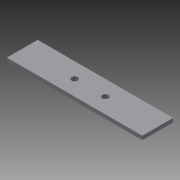
# Autodesk Inventor part: Cylinder Mount
Saved by Autodesk Inventor 2013 (Build 170138000, 138)
## iProperties
Created: 2013-01-26
Part Number: Cylinder Mount
Material: Generic
Document SubType Name: Sheet Metal
Designer: actoennies
Density: 1 g/cm^3
Sheet Metal Rule: Default
Mass: 23.7689 g
Surface Area: 175.75 cm^2
Volume: 23.7689 cm^3
Author: actoennies
Autodesk Inventor part; units mm, degrees
ref_plane "YZ Plane" through (0, 0, 0) normal (1, 0, 0) x (0, 1, 0)
ref_plane "XZ Plane" through (0, 0, 0) normal (0, 1, 0) x (-1, 0, 0)
ref_plane "XY Plane" through (0, 0, 0) normal (0, 0, 1) x (1, 0, 0)
sketch "Sketch13" plane through (0, 0, 0) normal (0, -1, 0) x (1, 0, 0)
  line L0 (0, 25.4) -> (-152.4, 25.4)
  line L1 (-152.4, 0) -> (-25.4, 0)
  line L2 (-25.4, -38.1) -> (0, -38.1)
  line L3 (-152.4, 0) -> (-152.4, -38.1)
  line L4 (-152.4, -38.1) -> (-127, -38.1)
  line L5 (-127, -38.1) -> (-127, 0)
  line L6 (-152.4, 25.4) -> (-152.4, 63.5)
  line L7 (-152.4, 63.5) -> (-127, 63.5)
  line L8 (-127, 63.5) -> (-127, 25.4)
  line L9 (0, 25.4) -> (0, 63.5)
  line L10 (0, 63.5) -> (-25.4, 63.5)
  line L11 (-25.4, 63.5) -> (-25.4, 25.4)
  circle A0 centre (-139.7, 50.8) radius 3.3782
  circle A1 centre (-139.7, -25.4) radius 3.3782
  circle A2 centre (-12.7, 50.8) radius 3.3782
  point P0 (0, 0)
  dimension "d73" = 25.4
  dimension "d74" = 38.1
  dimension "d75" = 25.4
  dimension "d76" = 38.1
  dimension "d77" = 25.4
  dimension "d78" = 6.7564
  dimension "d79" = 6.7564
  dimension "d80" = 6.7564
  dimension "d81" = 12.7
  dimension "d82" = 12.7
  dimension "d83" = 12.7
  dimension "d84" = 12.7
  dimension "d85" = 12.7
  dimension "d86" = 12.7
  dimension "d87" = 38.1
  measures "d73" distance of L3.end L4.end
  measures "d74" distance of L0.end L6.end
  measures "d75" distance of L6.end L7.end
  measures "d76" distance of L0.start L9.end
  measures "d77" distance of L9.end L10.end
  measures "d78" diameter of A0
  measures "d79" diameter of A1
  measures "d80" diameter of A2
  measures "d81" distance from line of L10 A2.centre
  measures "d82" distance from line of L9 A2.centre
  measures "d83" distance from line of L7 A0.centre
  measures "d84" distance from line of L8 A0.centre
  measures "d85" distance from line of L5 A1.centre
  measures "d86" distance from line of L4 A1.centre
  measures "d87" distance of L4.end L5.end
sketch "Sketch1" plane through (0, 0, 0) normal (0, 1, 0) x (-1, 0, 0)
  line L0 (0, 0) -> (0, 25.4)
  line L1 (0, 25.4) -> (152.4, 25.4)
  line L2 (152.4, 25.4) -> (152.4, 0)
  line L3 (152.4, 0) -> (25.4, 0)
  line L4 (0, 0) -> (0, -38.1)
  line L5 (0, -38.1) -> (25.4, -38.1)
  line L6 (25.4, -38.1) -> (25.4, 0)
  dimension "d0" = 25.4
  dimension "d1" = 152.4
  dimension "d58" = 38.1
  dimension "d59" = 25.4
  constraints: 14 end point, 4 perpendicular, 2 parallel, 1 vertical
  measures "d0" distance of L0.start L0.end
  measures "d1" distance of L0.end L1.end
  measures "d58" distance of L0.start L4.end
  measures "d59" distance of L4.end L5.end
extrude "Plate1" add sketch "Sketch1" along normal blind 3.175
sketch "Sketch5" plane through (0, 0, 0) normal (0, -1, 0) x (1, 0, 0)
  line L0 (0, 25.4) -> (-152.4, 25.4) projected
  line L1 (-152.4, 0) -> (-25.4, 0) projected
  circle A0 centre (-68.58, 12.7) radius 2.54
  circle A1 centre (-43.18, 12.7) radius 2.54
  line L2 (0, -38.1) -> (0, 25.4) projected
  line L3 (-152.4, 25.4) -> (-152.4, 0) projected
  line L4 (-55.88, 0) -> (-55.88, 25.4)
  point P0 (0, 0)
  dimension "d33" = 5.08
  dimension "d34" = 5.08
  dimension "d35" = 25.4
  dimension "d55" = 12.7
  dimension "d56" = 12.7
  dimension "d57" = 55.88
  constraints: 2 centre point, 2 end point, 2 point on line, 1 parallel
  measures "d33" diameter of A0
  measures "d34" diameter of A1
  measures "d35" distance of A1.centre A0.centre
  measures "d55" distance from line of A1.centre L4
  measures "d56" distance from line of A0.centre L4
  measures "d57" distance between parallel lines of L2 L4
extrude "Cut1" cut sketch "Sketch5" against normal blind 3.175 contours A0 | A1
sketch "Sketch10" plane through (0, 0, 0) normal (0, -1, 0) x (1, 0, 0)
  line L0 (0, -38.1) -> (0, 25.4) projected
  line L1 (-152.4, 25.4) -> (-152.4, 0) projected
  line L2 (-152.4, 0) -> (-25.4, 0) projected
  line L3 (-25.4, -38.1) -> (0, -38.1) projected
  circle A0 centre (-139.7, 12.7) radius 3.3782
  circle A1 centre (-12.7, -25.4) radius 3.3782
  point P0 (0, 0)
  dimension "d60" = 6.7564
  dimension "d61" = 12.7
  dimension "d62" = 12.7
  dimension "d63" = 6.7564
  dimension "d64" = 12.7
  dimension "d65" = 12.7
  constraints: 2 centre point
  measures "d60" diameter of A0
  measures "d61" distance from line of L1 A0.centre
  measures "d62" distance from line of L2 A0.centre
  measures "d63" diameter of A1
  measures "d64" distance from line of L0 A1.centre
  measures "d65" distance from line of L3 A1.centre
extrude "Cut6" cut sketch "Sketch10" against normal blind 3.175
sketch "Sketch12" plane through (0, 0, 0) normal (0, -1, 0) x (1, 0, 0)
  circle A0 centre (-12.7, 12.7) radius 3.3782
  point P0 (0, 0)
  constraints: 1 centre point
extrude "Cut7" cut sketch "Sketch12" against normal blind 3.175
sheet face with bend "Face2" sketch "Sketch13" thickness 3.175 toward (0, 1, 0) bend radius 3.175 relief straight relief width 3.175 relief depth 1.5875
bend "Bend4"
equation "\"d37\" = Thickness"
equation "\"d66\" = Thickness"
equation "\"d71\" = Thickness"
equation "\"d88\" = BendRadius"
equation "\"d89\" = BendReliefWidth"
equation "\"d91\" = MinimumRemnant"
equation "\"d90\" = BendReliefDepth"
equation "\"d92\" = BendRadius"
equation "\"BendRadius\" = Thickness"
equation "\"BendReliefWidth\" = Thickness"
equation "\"BendReliefDepth\" = 0.5 * Thickness"
equation "\"CornerReliefSize\" = 4 * Thickness"
equation "\"MinimumRemnant\" = 2 * Thickness"
equation "\"TransitionRadius\" = BendRadius"
equation "\"JacobiRadiusSize\" = BendRadius"
equation "\"GapSize\" = Thickness"
equation "\"d2\" = BendRadius"
equation "\"Thickness\" = 3.175"
body "Solid1"
